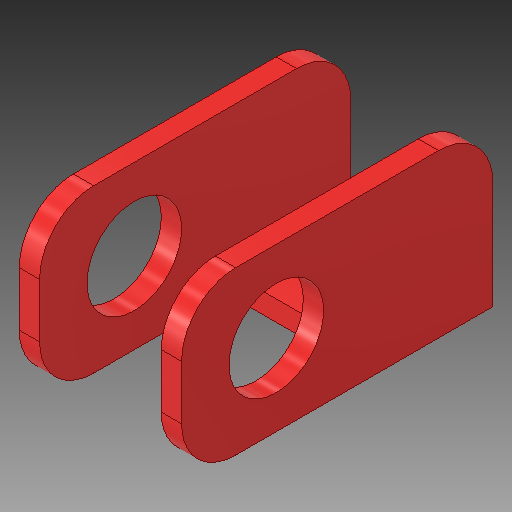
# Autodesk Inventor part: top pully bracket
Saved by Autodesk Inventor 2017 SP1 (Build 210196100, 196)
## iProperties
Created: 2018-01-20
Part Number: top pully bracket
Material: Aluminum 6061
Document SubType Name: Modeling
Designer: Ben
Density: 2.7 g/cm^3
Appearance: Light Red
Mass: 68.3621 g
Surface Area: 135.63 cm^2
Volume: 25.3193 cm^3
Author: Ben
Autodesk Inventor part; units mm, degrees
ref_plane "YZ Plane" through (0, 0, 0) normal (1, 0, 0) x (0, 1, 0)
ref_plane "XZ Plane" through (0, 0, 0) normal (0, 1, 0) x (-1, 0, 0)
ref_plane "XY Plane" through (0, 0, 0) normal (0, 0, 1) x (1, 0, 0)
sketch "Sketch1" plane through (0, 0, 0) normal (0, 0, 1) x (1, 0, 0)
  line L0 (-19.05, 38.1) -> (-14.2875, 38.1)
  line L1 (-14.2875, 38.1) -> (-14.2875, 4.7625)
  line L2 (-14.2875, 4.7625) -> (14.2875, 4.7625)
  line L3 (14.2875, 4.7625) -> (14.2875, 38.1)
  line L4 (14.2875, 38.1) -> (19.05, 38.1)
  line L5 (19.05, 38.1) -> (19.05, 0)
  line L6 (19.05, 0) -> (-19.05, 0)
  line L7 (-19.05, 0) -> (-19.05, 38.1)
  line L8 (0, 0) -> (0, 4.7625) construction
  dimension "d0" = 4.7625
  dimension "d2" = 38.1
  dimension "d3" = 38.1
  constraints: 18 end point, 5 perpendicular, 2 equal length, 2 horizontal, 2 midpoint, 2 point on line, 1 coincident
  measures "d0" distance of L3.end L4.end
  measures "d2" distance between parallel lines of L6 L4
  measures "d3" distance between parallel lines of L7 L5
extrude "Extrusion1" add sketch "Sketch1" along normal blind 73.025
sketch "Sketch2" plane through (-14.2875, 4.7625, 0) normal (0, 1, 0) x (1, 0, 0)
  line L0 (23.8125, -23.8125) -> (4.7625, -23.8125) construction
  line L1 (4.7625, -23.8125) -> (4.7625, -4.7625) construction
  line L2 (4.7625, -4.7625) -> (23.8125, -4.7625) construction
  line L3 (23.8125, -4.7625) -> (23.8125, -23.8125) construction
  line L4 (23.8125, -23.8125) -> (4.7625, -4.7625) construction
  line L5 (4.7625, -23.8125) -> (23.8125, -4.7625) construction
  circle A0 centre (4.7625, -4.7625) radius 2.54
  circle A1 centre (4.7625, -23.8125) radius 2.54
  circle A2 centre (23.8125, -4.7625) radius 2.54
  circle A3 centre (23.8125, -23.8125) radius 2.54
  line L6 (0, 0) -> (0, -73.025) projected
  line L7 (28.575, 0) -> (28.575, -73.025) projected
  line L8 (0, -73.025) -> (28.575, -73.025)
  line L9 (28.575, -73.025) -> (28.575, -28.575)
  line L10 (28.575, -28.575) -> (0, -28.575)
  line L11 (0, -28.575) -> (0, -73.025)
  line L12 (14.2875, -4.7625) -> (14.2875, 0) construction
  point P0 (14.2875, -14.2875)
  dimension "d6" = 5.08
  dimension "d7" = 19.05
  dimension "d8" = 19.05
  dimension "d10" = 14.2875
  dimension "d21" = 4.7625
  dimension "d22" = 4.7625
  constraints: 22 end point, 4 centre point, 4 coincident, 4 parallel, 3 equal radius, 3 midpoint, 2 horizontal, 2 perpendicular, 1 point on line, 1 vertical
  measures "d6" diameter of A0
  measures "d7" distance of L0.end L1.end
  measures "d8" distance of L1.end L2.end
  measures "d10" distance from line of L10 point (14.287, -14.288)
  measures "d21" distance from line of L12.end L2
  measures "d22" distance between parallel lines of L6 L1
extrude "Extrusion2" cut sketch "Sketch2" against normal through all
sketch "Sketch3" plane through (19.05, 0, 0) normal (1, 0, 0) x (0, 0, -1)
  circle A0 centre (-50.8, 19.05) radius 11.1125
  circle A1 centre (-50.8, 19.05) radius 17.4625 construction
  line L0 (-33.3375, 19.05) -> (-33.3375, -6.9181) construction
  line L1 (0, 0) -> (-73.025, 0) construction
  dimension "d15" = 34.925
  dimension "d13" = 22.225
  dimension "d14" = 19.05
  dimension "d16" = 33.3375
  constraints: 2 end point, 2 vertical, 1 centre point, 1 coincident, 1 horizontal alignment, 2 other
  measures "d13" diameter of A0
  measures "d14" vertical distance of L1.start A0.centre
  measures "d16" distance from line of L0 L1.start
extrude "Extrusion3" cut sketch "Sketch3" against normal through all
fillet "Fillet1" radius 12.7 6 edges at (16.6687, 38.1, 73.025) (-16.6687, 38.1, 73.025) (16.6687, 38.1, 0) (-16.6687, 38.1, 0) (-16.6688, 0, 73.025) (16.6688, 0, 73.025)
body "Solid1"
